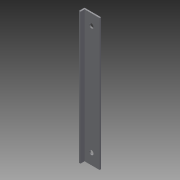
# Autodesk Inventor part: arm
Saved by Autodesk Inventor 2015 (Build 190159000, 159)
## iProperties
Created: 2016-01-20
Part Number: arm
Material: Generic
Document SubType Name: Modeling
Designer: 278648
Density: 1 g/cm^3
Appearance: Default
Author: 278648
Autodesk Inventor part; units mm, degrees
ref_plane "YZ Plane" through (0, 0, 0) normal (1, 0, 0) x (0, 1, 0)
ref_plane "XZ Plane" through (0, 0, 0) normal (0, 1, 0) x (-1, 0, 0)
ref_plane "XY Plane" through (0, 0, 0) normal (0, 0, 1) x (1, 0, 0)
sketch "Sketch1" plane through (0, 0, 0) normal (0, 1, 0) x (-1, 0, 0)
  line L0 (14.0408, 9.525) -> (10.8658, 9.525)
  line L1 (-24.0592, 0) -> (-24.0592, -3.175)
  line L2 (-24.0592, -3.175) -> (14.0408, -3.175)
  line L3 (14.0408, -3.175) -> (14.0408, 9.525)
  line L4 (10.8658, 9.525) -> (10.8658, 0)
  line L5 (10.8658, 0) -> (-24.0592, 0)
  point P0 (0, 0)
  dimension "d0" = 38.1
  dimension "d1" = 12.7
  dimension "d2" = 3.175
  dimension "d3" = 3.175
  constraints: 12 end point, 2 parallel, 2 perpendicular, 1 horizontal, 1 vertical
  measures "d0" distance between parallel lines of L3 L1
  measures "d1" distance between parallel lines of L0 L2
  measures "d2" distance between parallel lines of L5 L2
  measures "d3" distance between parallel lines of L3 L4
extrude "Extrusion1" add sketch "Sketch1" along normal blind 304.8
sketch "Sketch2" plane through (-10.8658, 0, 0) normal (0, 0, 1) x (1, 0, 0)
  circle A0 centre (15.875, 25.4) radius 4.9995
  line L0 (34.925, 0) -> (34.925, 304.8) projected
  line L1 (0, 0) -> (34.925, 0) projected
  circle A1 centre (15.875, 279.4) radius 4.9995
  line L2 (0, 304.8) -> (34.925, 304.8) projected
  point P0 (10.8658, 0)
  dimension "d6" = 19.05
  dimension "d7" = 25.4
  dimension "d8" = 19.05
  dimension "d9" = 25.4
  constraints: 2 centre point
  measures "d6" distance from line of A0.centre L0
  measures "d7" distance from line of A0.centre L1
  measures "d8" distance from line of L0 A1.centre
  measures "d9" distance from line of L2 A1.centre
extrude "Extrusion2" cut sketch "Sketch2" against normal through all
equation "\"d10\" = d7"
body "Solid1"
